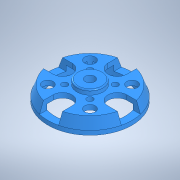
# Autodesk Inventor part: Top
Saved by Autodesk Inventor 2022 (Build 260153000, 153)
## iProperties
Created: 2022-07-28
Part Number: Top
Material: Stainless Steel
Document SubType Name: Modeling
Designer: Nathan Cai
Density: 8 g/cm^3
Appearance: Cyan
Author: Nathan Cai
Autodesk Inventor part; units mm, degrees
ref_plane "YZ Plane" through (0, 0, 0) normal (1, 0, 0) x (0, 1, 0)
ref_plane "XZ Plane" through (0, 0, 0) normal (0, 1, 0) x (-1, 0, 0)
ref_plane "XY Plane" through (0, 0, 0) normal (0, 0, 1) x (1, 0, 0)
sketch "Sketch1" plane through (0, 0, 0) normal (0, 0, 1) x (1, 0, 0)
  line L0 (0, 0) -> (17.6, 0)
  line L1 (17.6, 0) -> (17.6, 6)
  line L2 (17.6, 6) -> (0, 6)
  line L3 (0, 6) -> (0, 0) construction
  line L4 (0, 6) -> (5.5, 6)
  line L5 (5.5, 6) -> (5.5, 8)
  line L6 (5.5, 8) -> (0, 8)
  line L7 (0, 8) -> (0, 6) construction
  line L8 (16, 6) -> (16, 0) construction
  line L9 (16, 6) -> (17.6, 1.75)
  line L10 (0, 0) -> (2, 0)
  line L11 (2, 0) -> (2, 8)
  line L12 (2, 8) -> (0, 8)
  line L13 (0, 8) -> (0, 0) construction
  dimension "d0" = 17.6
  dimension "d1" = 6
  dimension "d2" = 5.5
  dimension "d3" = 2
  dimension "d4" = 16
  dimension "d5" = 1.75
  dimension "d6" = 2
  constraints: 28 end point, 6 parallel, 4 perpendicular, 4 point on line, 3 horizontal
  measures "d0" distance of L2.end L1.end
  measures "d1" distance between parallel lines of L0 L2
  measures "d2" distance of L6.end L5.end
  measures "d3" distance of L5.end L4.end
  measures "d4" distance between parallel lines of L3 L8
  measures "d5" distance from line of L0 L9.end
  measures "d6" distance of L12.end L11.end
revolve "Revolution1" add sketch "Sketch1" angle 360 about axis through (0, 8, 0) along (0, -1, 0) contours L11 L2 L9 L1 L0 | L11 L6 L5 L2
sketch "Sketch2" plane through (0, 6, 0) normal (0, 1, 0) x (1, 0, 0)
  arc A0 (-11.5, -4) -> (-11.5, 4) centre (-11.5, 0) ccw
  circle A1 centre (0, 0) radius 11.5 construction
  line L0 (-11.5, 0) -> (0, 0) construction
  line L1 (-11.5, -4) -> (-21.025, -4)
  line L2 (-21.025, -4) -> (-21.025, 4)
  line L3 (-21.025, 4) -> (-11.5, 4)
  line L4 (-11.5, 4) -> (-11.5, -4) construction
  circle A2 centre (0, 0) radius 2 projected
  circle A3 centre (0, 0) radius 7.5 construction
  circle A4 centre (0, 0) radius 12.5 construction
  line L5 (0, 0) -> (-8.8388, 8.8388) construction
  circle A5 centre (-5.3033, 5.3033) radius 1.25
  circle A6 centre (-8.8388, 8.8388) radius 2.25
  line L6 (-4, -11.5) -> (4, -11.5) construction
  line L7 (4, -11.5) -> (4, -21.025)
  line L8 (4, -21.025) -> (-4, -21.025)
  line L9 (-4, -21.025) -> (-4, -11.5)
  arc A7 (4, -11.5) -> (-4, -11.5) centre (0, -11.5) ccw
  circle A8 centre (-5.3033, -5.3033) radius 1.25
  circle A9 centre (-8.8388, -8.8388) radius 2.25
  line L10 (11.5, -4) -> (11.5, 4) construction
  line L11 (11.5, 4) -> (21.025, 4)
  line L12 (21.025, 4) -> (21.025, -4)
  line L13 (21.025, -4) -> (11.5, -4)
  arc A10 (11.5, 4) -> (11.5, -4) centre (11.5, 0) ccw
  circle A11 centre (5.3033, -5.3033) radius 1.25
  circle A12 centre (8.8388, -8.8388) radius 2.25
  line L14 (4, 11.5) -> (-4, 11.5) construction
  line L15 (-4, 11.5) -> (-4, 21.025)
  line L16 (-4, 21.025) -> (4, 21.025)
  line L17 (4, 21.025) -> (4, 11.5)
  arc A13 (-4, 11.5) -> (4, 11.5) centre (0, 11.5) ccw
  circle A14 centre (5.3033, 5.3033) radius 1.25
  circle A15 centre (8.8388, 8.8388) radius 2.25
  dimension "d9" = 23
  dimension "d11" = 15
  dimension "d12" = 25
  dimension "d8" = 8
  dimension "d10" = 9.525
  dimension "d13" = 45
  dimension "d14" = 2.5
  dimension "d15" = 4.5
  dimension "d18" = 360
  constraints: 36 end point, 12 centre point, 8 point on circle, 7 coincident, 2 horizontal, 2 parallel, 2 tangent, 1 horizontal alignment, 1 perpendicular, 1 point on line, 69 other
  measures "d8" diameter of A0
  measures "d10" distance of L2.end L3.end
  measures "d13" angle of L0 L5
  measures "d14" diameter of A5
  measures "d15" diameter of A6
extrude "Extrusion1" cut sketch "Sketch2" against normal blind 4.25
sketch "Sketch3" plane through (0, 0, 0) normal (0, -1, 0) x (1, 0, 0)
  circle A0 centre (0, 0) radius 2
  arc A1 (17.1394, 4) -> (4, 17.1394) centre (0, 0) ccw projected
  circle A2 centre (0, 0) radius 17.6
  circle A3 centre (0, 0) radius 14.6
  circle A4 centre (0, 0) radius 4
  dimension "d22" = 3
  dimension "d23" = 8
  constraints: 3 centre point, 3 coincident, 3 other
  measures "d23" diameter of A4
extrude "Extrusion2" cut sketch "Sketch3" against normal blind 4 contours A3
chamfer "Chamfer1" distance 4 angle 20 1 edges at (-4, 4, 0) measured on face at (3.987, 2.6667, -0.3219)
fillet "Fillet1" radius 0.5 1 edges at (-5.5, 8, 0)
body "Solid1"
